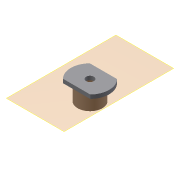
# Autodesk Inventor part: ECoG_holder_cap
Saved by Autodesk Inventor 2014 (Build 180170000, 170)
## iProperties
Created: 2016-07-27
Part Number: ECoG_holder_cap
Material: Generic
Document SubType Name: Modeling
Designer: Camilo
Density: 1 g/cm^3
Appearance: Default
Author: Camilo
Autodesk Inventor part; units mm, degrees
ref_plane "YZ Plane" through (0, 0, 0) normal (1, 0, 0) x (0, 1, 0)
ref_plane "XZ Plane" through (0, 0, 0) normal (0, 1, 0) x (-1, 0, 0)
ref_plane "XY Plane" through (0, 0, 0) normal (0, 0, 1) x (1, 0, 0)
ref_plane "Work Plane1" through (0, 0, 0) normal (0, 0, 1) x (1, 0, 0)
sketch "Sketch1" plane through (0, 0, 0) normal (0, 0, 1) x (1, 0, 0)
  arc A0 (-11, 8.1244) -> (-11, -8.1244) centre (0, 0) ccw construction
  line L0 (-11, -8.1244) -> (-11, -24.74) construction
  line L1 (-11, -24.74) -> (11, -24.74) construction
  line L2 (11, -24.74) -> (11, -8.1244) construction
  arc A1 (11, -8.1244) -> (11, 8.1244) centre (0, 0) ccw construction
  line L3 (11, 24.74) -> (11, 8.1244) construction
  line L4 (-11, 24.74) -> (11, 24.74) construction
  line L5 (-11, 8.1244) -> (-11, 24.74) construction
  line L6 (-7.0828, 6.9741) -> (7.0828, 6.9741)
  line L7 (-7.0828, -6.9741) -> (7.0828, -6.9741)
  arc A2 (-7.0828, 6.9741) -> (-7.0828, -6.9741) centre (0, 0) ccw
  arc A3 (7.0828, -6.9741) -> (7.0828, 6.9741) centre (0, 0) ccw
  arc A4 (-3.5454, 3.44) -> (-3.5454, -3.44) centre (0, 0) ccw projected
  line L8 (-3.5454, 3.44) -> (-1.1656, 3.44) projected
  line L9 (-1.1656, 3.44) -> (-1.1656, 4.44) projected
  line L10 (-1.1656, 4.44) -> (-2.5, 4.44) projected
  line L11 (-2.5, 4.44) -> (-2.5, 5.44) projected
  line L12 (-2.5, 5.44) -> (2.5, 5.44) projected
  line L13 (2.5, 5.44) -> (2.5, 4.44) projected
  line L14 (2.5, 4.44) -> (1.1656, 4.44) projected
  line L15 (1.1656, 4.44) -> (1.1656, 3.44) projected
  line L16 (1.1656, 3.44) -> (3.5454, 3.44) projected
  arc A5 (3.5454, -3.44) -> (3.5454, 3.44) centre (0, 0) ccw projected
  line L17 (1.1656, -3.44) -> (3.5454, -3.44) projected
  line L18 (1.1656, -4.44) -> (1.1656, -3.44) projected
  line L19 (1.1656, -4.44) -> (2.5, -4.44) projected
  line L20 (2.5, -4.44) -> (2.5, -5.44) projected
  line L21 (2.5, -5.44) -> (-2.5, -5.44) projected
  line L22 (-2.5, -5.44) -> (-2.5, -4.44) projected
  line L23 (-1.1656, -4.44) -> (-2.5, -4.44) projected
  line L24 (-1.1656, -3.44) -> (-1.1656, -4.44) projected
  line L25 (-3.5454, -3.44) -> (-1.1656, -3.44) projected
  point P0 (0, 0)
  constraints: 4 end point, 4 point on circle, 2 centre point, 1 coincident
extrude "Extrusion1" add sketch "Sketch1" along normal blind 2 contours L6 A3 L7 A2 | L8 L9 L10 L11 L12 L13 L14 L15 L16 A5 L17 L18 L19 L20 L21 L22 L23 L24 L25 A4
sketch "Sketch2" plane through (0, 0, 0) normal (0, 0, -1) x (-1, 0, 0)
  arc A0 (11, -8.1244) -> (11, 8.1244) centre (0, 0) ccw construction
  line L0 (11, -8.1244) -> (11, -24.74) construction
  line L1 (11, -24.74) -> (-11, -24.74) construction
  line L2 (-11, -24.74) -> (-11, -8.1244) construction
  arc A1 (-11, 8.1244) -> (-11, -8.1244) centre (0, 0) ccw construction
  line L3 (-11, 24.74) -> (-11, 8.1244) construction
  line L4 (11, 24.74) -> (-11, 24.74) construction
  line L5 (11, 8.1244) -> (11, 24.74) construction
  circle A2 centre (0, 0) radius 6.44
  circle A3 centre (0, 0) radius 4.44
  arc A4 (3.5454, -3.44) -> (3.5454, 3.44) centre (0, 0) ccw projected
  line L6 (3.5454, 3.44) -> (1.1656, 3.44) projected
  line L7 (1.1656, 3.44) -> (1.1656, 4.44) projected
  line L8 (1.1656, 4.44) -> (2.5, 4.44) projected
  line L9 (2.5, 4.44) -> (2.5, 5.44) projected
  line L10 (2.5, 5.44) -> (-2.5, 5.44) projected
  line L11 (-2.5, 5.44) -> (-2.5, 4.44) projected
  line L12 (-2.5, 4.44) -> (-1.1656, 4.44) projected
  line L13 (-1.1656, 4.44) -> (-1.1656, 3.44) projected
  line L14 (-1.1656, 3.44) -> (-3.5454, 3.44) projected
  arc A5 (-3.5454, 3.44) -> (-3.5454, -3.44) centre (0, 0) ccw projected
  line L15 (-1.1656, -3.44) -> (-3.5454, -3.44) projected
  line L16 (-1.1656, -4.44) -> (-1.1656, -3.44) projected
  line L17 (-1.1656, -4.44) -> (-2.5, -4.44) projected
  line L18 (-2.5, -4.44) -> (-2.5, -5.44) projected
  line L19 (-2.5, -5.44) -> (2.5, -5.44) projected
  line L20 (2.5, -5.44) -> (2.5, -4.44) projected
  line L21 (1.1656, -4.44) -> (2.5, -4.44) projected
  line L22 (1.1656, -3.44) -> (1.1656, -4.44) projected
  line L23 (3.5454, -3.44) -> (1.1656, -3.44) projected
  dimension "d6" = 2
  constraints: 2 centre point, 2 coincident
  measures "d6" radial gap between concentric circles of A2 A3
extrude "Extrusion2" add sketch "Sketch2" along normal blind 8 contours A2 | A3 L6 A4 L23 | A3 L13 L12 L11 L10 L9 L8 L7 | L22 L21 L20 L19 L18 L17 L16 A3 | A3 L15 A5 L14
sketch "Sketch3" plane through (0, 0, 2) normal (0, 0, 1) x (1, 0, 0)
  arc A0 (7.0828, -6.9741) -> (7.0828, 6.9741) centre (0, 0) ccw projected
  circle A1 centre (0, 0) radius 2
  constraints: 1 centre point, 1 coincident
extrude "Extrusion3" cut sketch "Sketch3" against normal through all
body "Solid1"
